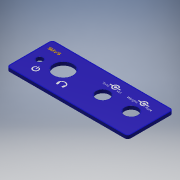
# Autodesk Inventor part: frontPlate
Saved by Autodesk Inventor 2016 (Build 200138000, 138)
## iProperties
Created: 2017-03-04
Part Number: frontPlate
Material: Generic
Document SubType Name: Modeling
Designer: Tyler
Density: 1 g/cm^3
Appearance: Default
Author: Tyler
Autodesk Inventor part; units mm, degrees
ref_plane "YZ Plane" through (0, 0, 0) normal (1, 0, 0) x (0, 1, 0)
ref_plane "XZ Plane" through (0, 0, 0) normal (0, 1, 0) x (-1, 0, 0)
ref_plane "XY Plane" through (0, 0, 0) normal (0, 0, 1) x (1, 0, 0)
sketch "Sketch1" plane through (0, 0, 0) normal (0, 0, 1) x (1, 0, 0)
  line L0 (-29.75, -11.25) -> (29.75, -11.25)
  line L1 (29.75, -11.25) -> (29.75, 11.25)
  line L2 (29.75, 11.25) -> (-29.75, 11.25)
  line L3 (-29.75, 11.25) -> (-29.75, -11.25)
  line L4 (-29.75, -11.25) -> (29.75, 11.25) construction
  line L5 (29.75, -11.25) -> (-29.75, 11.25) construction
  point P0 (0, 0)
  dimension "d0" = 59.5
  dimension "d1" = 22.5
  constraints: 12 end point, 2 midpoint, 2 parallel, 1 horizontal, 1 perpendicular
  measures "d0" distance of L2.end L1.end
  measures "d1" distance of L0.end L1.end
extrude "Extrusion1" add sketch "Sketch1" against normal blind 1.6
fillet "Fillet1" radius 1.5 4 edges at (29.75, 11.25, -0.8) (29.75, -11.25, -0.8) (-29.75, 11.25, -0.8) (-29.75, -11.25, -0.8)
sketch "Sketch2" plane through (0, 0, 0) normal (0, 0, 1) x (1, 0, 0)
  circle A0 centre (-14.379, 1.26) radius 4.75
  line L0 (-28.25, -11.25) -> (28.25, -11.25) projected
  line L1 (-29.75, 9.75) -> (-29.75, -9.75) projected
  point P0 (0, 0)
  dimension "d5" = 9.5
  dimension "d15" = 12.51
  dimension "d16" = 15.371
  constraints: 1 centre point
  measures "d5" diameter of A0
  measures "d15" distance from line of L0 A0.centre
  measures "d16" distance from line of A0.centre L1
extrude "Extrusion2" cut sketch "Sketch2" against normal through all
sketch "Sketch3" plane through (0, 0, 0) normal (0, 0, 1) x (1, 0, 0)
  line L0 (-28.25, -11.25) -> (28.25, -11.25) projected
  circle A0 centre (5.985, 0.26) radius 3.25
  circle A1 centre (19.955, 0.26) radius 3.25
  point P0 (0, 0)
  dimension "d8" = 6.5
  dimension "d9" = 13.97
  dimension "d10" = 11.51
  dimension "d11" = 5.985
  dimension "d14" = 11.51
  constraints: 2 centre point, 1 equal radius
  measures "d8" diameter of A0
  measures "d9" distance of A1.centre A0.centre
  measures "d10" distance from line of L0 A1.centre
  measures "d11" horizontal distance of point (0, 0) A0.centre
  measures "d14" distance from line of L0 A0.centre
extrude "Extrusion3" cut sketch "Sketch3" against normal through all
sketch "Sketch4" plane through (0, 0, 0) normal (0, 0, 1) x (1, 0, 0)
  line L0 (-28.25, -11.25) -> (28.25, -11.25) projected
  line L1 (-29.75, 9.75) -> (-29.75, -9.75) projected
  circle A0 centre (-24.539, -0.14) radius 1.55
  point P0 (0, 0)
  point P1 (-28.349, -5.24)
  dimension "d17" = 6.01
  dimension "d18" = 1.401
  dimension "d19" = 3.1
  dimension "d20" = 3.81
  dimension "d21" = 5.1
  constraints: 1 centre point
  measures "d17" distance from line of L0 point (-28.349, -5.24)
  measures "d18" distance from line of L1 point (-28.349, -5.24)
  measures "d19" diameter of A0
  measures "d20" horizontal distance of A0.centre point (-28.349, -5.24)
  measures "d21" vertical distance of point (-28.349, -5.24) A0.centre
extrude "Extrusion4" cut sketch "Sketch4" against normal through all
sketch "Sketch5" plane through (0, 0, 0) normal (0, 0, 1) x (1, 0, 0)
  line L0 (-29.75, 11.25) -> (29.75, 11.25) construction
  line L1 (29.75, 11.25) -> (29.75, -11.2473) construction
  line L2 (29.75, -11.2473) -> (-29.75, -11.2473) construction
  line L3 (-29.75, -11.2473) -> (-29.75, 11.25) construction
  line L4 (28.25, 11.25) -> (-28.25, 11.25) projected
  line L5 (-29.75, 9.75) -> (-29.75, -9.75) projected
  line L6 (29.75, -9.75) -> (29.75, 9.75) projected
  point P0 (0, 0)
  constraints: 3 collinear, 2 other
decal "Decal1"
equation "\"d14\" = d10"
body "Solid1"
